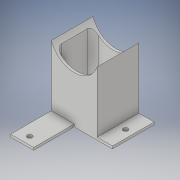
# Autodesk Inventor part: DPLX_P016_Spark_Gap_Camera_Shroud
Saved by Autodesk Inventor 2018 (Build 220112000, 112)
## iProperties
Created: 2018-06-12
Part Number: DPLX_P016_Spark_Gap_Camera_Shroud
Material: Generic
Document SubType Name: Modeling
Designer: DPLXuser
Density: 1 g/cm^3
Appearance: Default
Author: DPLXuser
Autodesk Inventor part; units mm, degrees
ref_plane "YZ Plane" through (0, 0, 0) normal (1, 0, 0) x (0, 1, 0)
ref_plane "XZ Plane" through (0, 0, 0) normal (0, 1, 0) x (-1, 0, 0)
ref_plane "XY Plane" through (0, 0, 0) normal (0, 0, 1) x (1, 0, 0)
sketch "Sketch1" plane through (0, 0, 0) normal (0, 1, 0) x (-1, 0, 0)
  line L0 (-14.3278, -13.0048) -> (14.3278, -13.0048)
  line L1 (14.3278, -13.0048) -> (14.3278, 13.0048)
  line L2 (14.3278, 13.0048) -> (-14.3278, 13.0048)
  line L3 (-14.3278, 13.0048) -> (-14.3278, -13.0048)
  line L4 (-14.3278, -13.0048) -> (14.3278, 13.0048) construction
  line L5 (14.3278, -13.0048) -> (-14.3278, 13.0048) construction
  point P0 (0, 0)
  dimension "d0" = 28.6557
  dimension "d1" = 26.0096
  constraints: 12 end point, 2 midpoint, 2 parallel, 1 horizontal, 1 perpendicular
  measures "d0" distance of L2.end L1.end
  measures "d1" distance of L1.end L0.end
extrude "Extrusion1" add sketch "Sketch1" along normal blind 40.1371
shell "Shell1" thickness 1.5875 removed faces 2 at (4.7759, 0, 4.3349) at (4.7759, 40.1371, 4.3349)
sketch "Sketch2" plane through (0, 0, 0) normal (0, 0, 1) x (1, 0, 0)
  line L0 (0, 0) -> (0, 44.45)
  circle A0 centre (0, 44.45) radius 15.113
  dimension "d5" = 44.45
  dimension "d6" = 30.226
  constraints: 2 end point, 1 centre point, 1 coincident, 1 vertical
  measures "d5" distance of L0.start L0.end
  measures "d6" diameter of A0
extrude "Extrusion2" cut sketch "Sketch2" along normal mid plane 39.1617
sketch "Sketch4" plane through (-14.3278, 0, -13.0048) normal (-1, 0, 0) x (0, 0, 1)
  line L0 (26.0096, 0) -> (26.0096, 39.6421) projected
  line L1 (0, 0) -> (26.0096, 0)
  line L2 (26.0096, 0) -> (26.0096, 3.175)
  line L3 (26.0096, 3.175) -> (0, 3.175)
  line L4 (0, 3.175) -> (0, 0)
  point P0 (13.0048, 0)
  constraints: 8 end point, 2 parallel, 1 horizontal, 1 perpendicular
extrude "Extrusion4" [suppressed]
sketch "Sketch5" plane through (0, 0, 0) normal (0, -1, 0) x (1, 0, 0)
  line L0 (12.7403, 11.4173) -> (-12.7403, 11.4173)
  line L1 (-12.7403, 11.4173) -> (-12.7403, -11.4173)
  line L2 (-12.7403, -11.4173) -> (12.7403, -11.4173)
  line L3 (12.7403, -11.4173) -> (12.7403, 11.4173)
  point P0 (0, 0)
  constraints: 8 end point, 2 parallel, 1 horizontal, 1 perpendicular
extrude "Extrusion5" add sketch "Sketch5" against normal blind 3.175
sketch "Sketch6" plane through (0, 0, 0) normal (0, -1, 0) x (1, 0, 0)
  line L0 (0, 0) -> (-1.4907, 0)
  circle A0 centre (-1.4907, 0) radius 6.35
  dimension "d22" = 1.4907
  dimension "d23" = 12.7
  constraints: 2 end point, 1 centre point, 1 coincident, 1 horizontal
  measures "d22" distance of L0.start L0.end
  measures "d23" diameter of A0
extrude "Extrusion6" cut sketch "Sketch6" against normal blind 3.175
fillet "Fillet1" radius 3.175 4 edges at (-12.7403, 19.7478, -11.4173) (-12.7403, 19.7478, 11.4173) (12.7403, 19.7478, 11.4173) (12.7403, 19.7478, -11.4173)
sketch "Sketch11" plane through (14.3278, 0, 13.0048) normal (1, 0, 0) x (0, 0, -1)
  line L0 (0, 0) -> (0, 39.6421) projected
  line L1 (26.0096, 0) -> (26.0096, 39.6421) projected
  line L2 (0, 0) -> (26.0096, 0)
  line L3 (26.0096, 0) -> (26.0096, 1.5875)
  line L4 (26.0096, 1.5875) -> (0, 1.5875)
  line L5 (0, 1.5875) -> (0, 0)
  point P0 (13.0048, 0)
  dimension "d36" = 1.5875
  constraints: 8 end point, 2 parallel, 1 horizontal, 1 perpendicular, 1 point on line
  measures "d36" distance of L3.end L2.end
extrude "Extrusion11" add sketch "Sketch11" along normal blind 9.525
sketch "Sketch12" plane through (0, 44.45, -13.0048) normal (0, 0, -1) x (-1, 0, 0)
  line L0 (-23.8528, -44.45) -> (14.3278, -44.45) projected
  line L1 (0, -44.45) -> (0, -42.8625) projected
  line L2 (14.3278, -44.45) -> (0, -44.45)
  line L3 (0, -44.45) -> (0, -42.8625)
  line L4 (0, -42.8625) -> (14.3278, -42.8625)
  line L5 (14.3278, -42.8625) -> (14.3278, -44.45)
  dimension "d39" = 1.5875
  constraints: 8 end point, 2 parallel, 1 horizontal, 1 perpendicular
  measures "d39" distance of L2.end L1.end
extrude "Extrusion12" add sketch "Sketch12" along normal blind 9.525
sketch "Sketch13" plane through (0, 44.45, 13.0048) normal (0, 0, 1) x (1, 0, 0)
  point P0 (0, -44.45)
sketch "Sketch14" plane through (-14.3278, 0, 13.0048) normal (-1, 0, 0) x (0, 0, 1)
  point P0 (-13.0048, 0)
sketch "Sketch15" plane through (0, 44.45, 13.0048) normal (0, 0, 1) x (1, 0, 0)
  line L0 (-14.3278, -44.45) -> (23.8528, -44.45) projected
  line L1 (-14.3278, -44.45) -> (0, -44.45)
  line L2 (0, -44.45) -> (0, -42.8625)
  line L3 (0, -42.8625) -> (-14.3278, -42.8625)
  line L4 (-14.3278, -42.8625) -> (-14.3278, -44.45)
  point P0 (0, -44.45)
  dimension "d42" = 1.5875
  constraints: 8 end point, 2 parallel, 1 horizontal, 1 perpendicular
  measures "d42" distance of L2.end L1.end
extrude "Extrusion13" add sketch "Sketch15" along normal blind 25.4
sketch "Sketch16" plane through (-14.3278, 1.5875, -13.0048) normal (0, 1, 0) x (1, 0, 0)
  line L0 (14.3278, 0) -> (14.3278, 9.525) projected
  line L1 (0, -51.4096) -> (0, 9.525) projected
  line L2 (14.3278, 9.525) -> (0, 9.525) projected
  line L3 (14.3278, -26.0096) -> (14.3278, -51.4096) projected
  line L4 (38.1807, -26.0096) -> (38.1807, 0) projected
  line L5 (14.3278, -26.0096) -> (38.1807, -26.0096) projected
  line L6 (38.1807, 0) -> (14.3278, 0) projected
  line L7 (38.1807, 0) -> (33.4182, 0)
  circle A0 centre (7.1639, 4.7625) radius 1.524
  circle A1 centre (33.4182, -13.0048) radius 1.524
  circle A2 centre (7.1639, -46.6471) radius 1.524
  point P0 (14.3278, -13.0048)
  dimension "d45" = 4.7625
  dimension "d47" = 3.048
  dimension "d48" = 3.048
  dimension "d63" = 3.048
  constraints: 3 centre point, 2 end point, 1 horizontal
  measures "d45" distance of L4.end L7.end
  measures "d47" diameter of A0
  measures "d48" diameter of A1
  measures "d63" diameter of A2
extrude "Extrusion14" cut sketch "Sketch16" against normal blind 25.4
body "Solid1"
